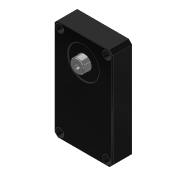
# Autodesk Inventor part: XM540_HOUSING_TOP
Saved by Autodesk Inventor 2019.4 (Build 234330000, 330)
## iProperties
Created: 2019-10-19
Part Number: XM540_HOUSING_TOP
Material: 一般
Document SubType Name: Modeling
Designer: y6tada
Density: 1 g/cm^3
Appearance: 滑らか - 黒
Author: y6tada
Autodesk Inventor part; units mm, degrees
ref_plane "YZ Plane" through (0, 0, 0) normal (1, 0, 0) x (0, 1, 0)
ref_plane "XZ Plane" through (0, 0, 0) normal (0, 1, 0) x (-1, 0, 0)
ref_plane "XY Plane" through (0, 0, 0) normal (0, 0, 1) x (1, 0, 0)
sketch "スケッチ1" plane through (0, 0, 0) normal (0, 0, 1) x (1, 0, 0)
  line L0 (-14.75, 13.75) -> (14.75, 13.75)
  line L1 (16.75, 11.75) -> (16.75, -42.75)
  line L2 (14.75, -44.75) -> (-14.75, -44.75)
  line L3 (-16.75, -42.75) -> (-16.75, 11.75)
  line L4 (-14.75, 13.75) -> (-16.75, 11.75)
  line L5 (14.75, 13.75) -> (16.75, 11.75)
  line L6 (16.75, -42.75) -> (14.75, -44.75)
  line L7 (-14.75, -44.75) -> (-16.75, -42.75)
  line L8 (0, 0) -> (0, -49.9081) construction
  circle A0 centre (0, 0) radius 13 construction
  line L9 (-13.5, 10.5) -> (13.5, 10.5) construction
  line L10 (13.5, 10.5) -> (13.5, -41.5) construction
  line L11 (13.5, -41.5) -> (-13.5, -41.5) construction
  line L12 (-13.5, -41.5) -> (-13.5, 10.5) construction
  circle A1 centre (-13.5, 10.5) radius 1.25
  circle A2 centre (13.5, 10.5) radius 1.25
  circle A3 centre (13.5, -41.5) radius 1.25
  circle A4 centre (-13.5, -41.5) radius 1.25
  circle A5 centre (0, 0) radius 4.2
  point P0 (-16.75, 13.75)
  point P1 (16.75, -44.75)
  point P2 (16.75, 13.75)
  point P3 (-16.75, -44.75)
  dimension "d0" = 2
  dimension "d1" = 2
  dimension "d2" = 2
  dimension "d3" = 2
  dimension "d4" = 2
  dimension "d5" = 2
  dimension "d6" = 2
  dimension "d7" = 2
  dimension "d8" = 33.5
  dimension "d9" = 26
  dimension "d10" = 13.75
  dimension "d11" = 58.5
  dimension "d24" = 27
  dimension "d25" = 10.5
  dimension "d26" = 52
  dimension "d27" = 2.5
  dimension "d31" = 8.4
  constraints: 26 end point, 8 point on line, 6 centre point, 6 coincident, 4 parallel, 3 equal radius, 2 horizontal, 2 perpendicular, 1 vertical, 2 other
  measures "d0" distance of L0.start point (-16.75, 13.75)
  measures "d1" distance of L3.end point (-16.75, 13.75)
  measures "d2" distance of L0.end point (16.75, 13.75)
  measures "d3" distance of L1.start point (16.75, 13.75)
  measures "d4" distance of L1.end point (16.75, -44.75)
  measures "d5" distance of L2.start point (16.75, -44.75)
  measures "d6" distance of L2.end point (-16.75, -44.75)
  measures "d7" distance of L3.start point (-16.75, -44.75)
  measures "d8" distance between parallel lines of L1 L3
  measures "d9" diameter of A0
  measures "d10" distance from line of L8.start L0
  measures "d11" distance between parallel lines of L2 L0
  measures "d24" distance of L9.start L9.end
  measures "d25" distance from line of A0.centre L9
  measures "d26" distance of L9.end L10.end
  measures "d27" diameter of A1
  measures "d31" diameter of A5
extrude "押し出し1" add sketch "スケッチ1" along normal blind 11.5
sketch "スケッチ2" plane through (0, 0, 11.5) normal (0, 0, 1) x (1, 0, 0)
  line L0 (-13.5, 10.5) -> (13.5, 10.5) construction
  line L1 (13.5, 10.5) -> (13.5, -41.5) construction
  line L2 (13.5, -41.5) -> (-13.5, -41.5) construction
  line L3 (-13.5, -41.5) -> (-13.5, 10.5) construction
  line L4 (0, 0) -> (0, 31.2445) construction
  circle A0 centre (13.5, 10.5) radius 2.4
  circle A1 centre (13.5, -41.5) radius 2.4
  circle A2 centre (-13.5, -41.5) radius 2.4
  circle A3 centre (-13.5, 10.5) radius 2.4
  dimension "d18" = 27
  dimension "d19" = 10.5
  dimension "d20" = 52
  dimension "d21" = 4.8
  constraints: 10 end point, 4 centre point, 4 coincident, 3 equal radius, 2 parallel, 1 horizontal, 1 perpendicular, 1 vertical, 1 other
  measures "d18" distance of L0.start L0.end
  measures "d19" distance from line of L0 L4.start
  measures "d20" distance of L0.end L1.end
  measures "d21" diameter of A0
extrude "押し出し2" cut sketch "スケッチ2" against normal blind 2.8
sketch "スケッチ3" plane through (0, 0, 11.5) normal (0, 0, 1) x (1, 0, 0)
  circle A0 centre (0, 0) radius 9
  dimension "d28" = 18
  constraints: 1 centre point, 1 coincident
  measures "d28" diameter of A0
extrude "押し出し3" cut sketch "スケッチ3" against normal blind 0.6
chamfer "面取り1" distance 0.2 angle 45 9 edges at (-9, 0, 11.5) (-15.75, -43.75, 0) (-16.75, -15.5, 0) (0, -44.75, 0) (15.75, -43.75, 0) (16.75, -15.5, 0) (15.75, 12.75, 0) (0, 13.75, 0) (-15.75, 12.75, 0)
chamfer "面取り2" distance 0.4 angle 45 8 edges at (-16.75, -15.5, 11.5) (-15.75, 12.75, 11.5) (0, 13.75, 11.5) (15.75, 12.75, 11.5) (16.75, -15.5, 11.5) (15.75, -43.75, 11.5) (0, -44.75, 11.5) (-15.75, -43.75, 11.5)
sketch "スケッチ4" plane through (0, 0, 0) normal (0, 1, 0) x (-1, 0, 0)
  line L0 (0, 0) -> (-1.5, 0) construction
  line L1 (-4, 0) -> (-4, 14.7)
  line L2 (-3.5, 15.2) -> (-1.75, 15.2)
  line L3 (0, 15.2) -> (0, 0) construction
  line L4 (-4, 14.7) -> (-3.5, 15.2)
  line L5 (-14.75, 11.5) -> (14.75, 11.5) construction
  line L6 (-1.5, 14.95) -> (-1.5, 0)
  line L7 (-1.5, 14.95) -> (-1.75, 15.2)
  line L8 (-1.5, 0) -> (-4, 0)
  point P0 (-4, 15.2)
  point P1 (-1.5, 15.2)
  point P2 (-1.5, 15.2)
  dimension "d32" = 0.5
  dimension "d33" = 0.5
  dimension "d34" = 8
  dimension "d35" = 3.7
  dimension "d45" = 3
  dimension "d46" = 0.25
  dimension "d47" = 0.25
  constraints: 16 end point, 7 point on line, 3 parallel, 2 horizontal, 2 perpendicular, 1 vertical
  measures "d32" distance of L1.end point (-4, 15.2)
  measures "d33" distance of L2.start point (-4, 15.2)
  measures "d34" diameter of L1 L3
  measures "d35" distance between parallel lines of L2 L5
  measures "d45" diameter of L6 L3
  measures "d46" distance of L6.start point (-1.5, 15.2)
  measures "d47" distance of L2.end point (-1.5, 15.2)
revolve "回転1" add sketch "スケッチ4" angle 360 about axis through (0, 0, 15.2) along (0, 0, -1)
equation "\"d1\" = d0"
equation "\"d2\" = d0"
equation "\"d3\" = d2"
equation "\"d4\" = d0"
equation "\"d5\" = d4"
equation "\"d6\" = d0"
equation "\"d7\" = d6"
equation "\"d33\" = d32"
equation "\"d47\" = d46"
